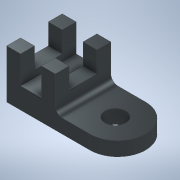
# Autodesk Inventor part: Saddle Bracket
Saved by Autodesk Inventor 2021.1 (Build 251245000, 245)
## iProperties
Created: 2021-05-10
Part Number: Saddle Bracket
Material: Iron, Cast
Document SubType Name: Modeling
Designer: as000166
Density: 7.15 g/cm^3
Appearance: Iron Gray
Mass: 669.768 g
Surface Area: 201.252 cm^2
Volume: 93.6739 cm^3
Author: as000166
Autodesk Inventor part; units mm, degrees
ref_plane "YZ Plane" through (0, 0, 0) normal (1, 0, 0) x (0, 1, 0)
ref_plane "XZ Plane" through (0, 0, 0) normal (0, 1, 0) x (-1, 0, 0)
ref_plane "XY Plane" through (0, 0, 0) normal (0, 0, 1) x (1, 0, 0)
sketch "Sketch1" plane through (0, 0, 0) normal (0, 0, 1) x (1, 0, 0)
  line L0 (0, 0) -> (0, 44.45)
  line L1 (0, 44.45) -> (12.7, 44.45)
  line L2 (0, 0) -> (76.2, 0)
  line L3 (76.2, 0) -> (76.2, 12.7)
  line L4 (76.2, 12.7) -> (50.8, 12.7)
  line L5 (44.45, 19.05) -> (44.45, 44.45)
  line L6 (44.45, 44.45) -> (31.75, 44.45)
  line L7 (31.75, 44.45) -> (31.75, 19.05)
  line L8 (12.7, 44.45) -> (12.7, 19.05)
  line L9 (12.7, 19.05) -> (31.75, 19.05)
  arc A0 (44.45, 19.05) -> (50.8, 12.7) centre (50.8, 19.05) ccw
  point P0 (44.45, 12.7)
  dimension "d0" = 44.45
  dimension "d1" = 12.7
  dimension "d2" = 76.2
  dimension "d3" = 12.7
  dimension "d4" = 31.75
  dimension "d5" = 31.75
  dimension "d6" = 12.7
  dimension "d7" = 25.4
  dimension "d8" = 25.4
  dimension "d9" = 19.05
  dimension "d26" = 6.35
  constraints: 20 end point, 6 perpendicular, 2 point on circle, 2 point on line, 2 tangent, 2 vertical, 1 centre point, 1 horizontal
  measures "d0" distance of L0.start L0.end
  measures "d1" distance of L0.end L1.end
  measures "d2" distance of L0.start L2.end
  measures "d3" distance of L2.end L3.end
  measures "d4" distance of L3.end point (44.45, 12.7)
  measures "d5" distance of point (44.45, 12.7) L5.end
  measures "d6" distance of L5.end L6.end
  measures "d7" distance of L6.end L7.end
  measures "d8" distance of L1.end L8.end
  measures "d9" distance of L8.end L7.end
  measures "d26" radius of A0
extrude "Base" add sketch "Sketch1" along normal mid plane 50.8
sketch "Sketch2" plane through (0, 0, 25.4) normal (0, -1, 0) x (1, 0, 0)
  line L0 (76.2, -50.8) -> (76.2, 0) projected
  circle A0 centre (76.2, -25.4) radius 25.4
  point P0 (0, -25.4)
  point P1 (76.2, 0)
  constraints: 1 midpoint, 3 other
extrude "Circle_EXT" add sketch "Sketch2" against normal up to surface (12.7 mm away) contours L0 A0 picked at (83.8282, -21.7265)
sketch "Sketch3" plane through (44.45, 12.7, 25.4) normal (0, 1, 0) x (1, 0, 0)
  point P0 (-44.45, 25.4)
  point P1 (29.7441, 25.1789)
hole "Hole1" at (74.1941, 12.7, 0.2211) direction (0, -1, 0) diameter 19.05 end through all
sketch "Sketch4" plane through (44.45, 12.7, 25.4) normal (1, 0, 0) x (0, 0, -1)
  line L0 (0, 31.75) -> (0, 6.35) projected
  line L1 (0, 31.75) -> (50.8, 31.75) projected
  line L2 (12.7, 31.75) -> (12.7, 12.7)
  line L3 (12.7, 12.7) -> (38.1, 12.7)
  line L4 (38.1, 12.7) -> (38.1, 31.75)
  point P0 (25.4, -12.7)
  dimension "d22" = 19.05
  dimension "d23" = 25.4
  constraints: 6 end point, 2 point on line, 1 horizontal, 1 perpendicular, 1 vertical
  measures "d22" distance of L2.start L2.end
  measures "d23" distance of L2.end L3.end
extrude "RECT_CUT" cut sketch "Sketch4" against normal through all
body "Solid1"
